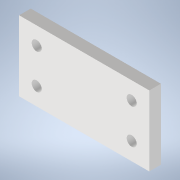
# Autodesk Inventor part: Muñeca2
Saved by Autodesk Inventor 2022 (Build 260153000, 153)
## iProperties
Created: 2021-09-13
Part Number: Muñeca2
Material: Generic
Document SubType Name: Modeling
Designer: Administrador
Density: 1 g/cm^3
Appearance: Default
Author: Administrador
Autodesk Inventor part; units mm, degrees
ref_plane "YZ Plane" through (0, 0, 0) normal (1, 0, 0) x (0, 1, 0)
ref_plane "XZ Plane" through (0, 0, 0) normal (0, 1, 0) x (-1, 0, 0)
ref_plane "XY Plane" through (0, 0, 0) normal (0, 0, 1) x (1, 0, 0)
sketch "Sketch1" plane through (0, 0, 0) normal (0, 0, 1) x (1, 0, 0)
  circle A0 centre (13, 16) radius 1.425
  circle A1 centre (13, 6.05) radius 1.425
  circle A2 centre (40, 6.05) radius 1.425
  circle A3 centre (40, 16) radius 1.425
  line L0 (45, 1.05) -> (8, 1.05)
  line L1 (8, 1.05) -> (8, 21)
  line L2 (8, 21) -> (45, 21)
  line L3 (45, 21) -> (45, 1.05)
  point P0 (0, 0)
  dimension "d24" = 9.95
  dimension "d27" = 9.95
  dimension "d31" = 5
  dimension "d32" = 5
  dimension "d33" = 5
  dimension "d34" = 5
  dimension "d40" = 5
  dimension "d41" = 5
  dimension "d42" = 5
  dimension "d43" = 27
  constraints: 8 end point, 4 centre point, 1 parallel
  measures "d24" distance of A0.centre A1.centre
  measures "d27" distance of A2.centre A3.centre
  measures "d31" distance from line of L0 A2.centre
  measures "d32" distance from line of L2 A0.centre
  measures "d33" distance from line of L1 A0.centre
  measures "d34" distance from line of A1.centre L0
  measures "d40" distance from line of L3 A2.centre
  measures "d41" distance from line of L3 A3.centre
  measures "d42" distance from line of L2 A3.centre
  measures "d43" distance of A0.centre A3.centre
extrude "Extrusion1" add sketch "Sketch1" along normal blind 3.3
body "Solid1"
